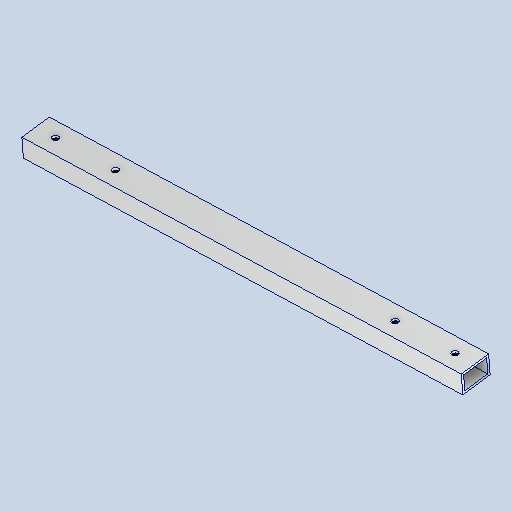
# Autodesk Inventor part: left_ASP
Saved by Autodesk Inventor 2024 (Build 280153000, 153)
## iProperties
Created: 2023-10-26
Part Number: left_ASP
Material: アルミニウム 6061
Document SubType Name: Modeling
Designer: jwith
Density: 2.7 g/cm^3
Appearance: アルミニウム - フラット
Mass: 32.0101 g
Surface Area: 199.643 cm^2
Volume: 11.8556 cm^3
Author: jwith
Autodesk Inventor part; units mm, degrees
ref_plane "YZ Plane" through (0, 0, 0) normal (1, 0, 0) x (0, 1, 0)
ref_plane "XZ Plane" through (0, 0, 0) normal (0, 1, 0) x (-1, 0, 0)
ref_plane "XY Plane" through (0, 0, 0) normal (0, 0, 1) x (1, 0, 0)
sketch "スケッチ1" plane through (0, 0, 0) normal (0, 1, 0) x (-1, 0, 0)
  line L0 (0, 0) -> (-15, 0)
  line L1 (-15, 0) -> (-15, -10)
  line L2 (-15, -10) -> (0, -10)
  line L3 (0, -10) -> (0, 0)
  dimension "d0" = 15
  dimension "d1" = 10
  constraints: 8 end point, 2 parallel, 1 horizontal, 1 perpendicular
  measures "d0" distance of L1.end L2.end
  measures "d1" distance of L2.end L0.start
extrude "押し出し1" add sketch "スケッチ1" against normal blind 220
shell "シェル1" thickness 1.2 removed faces 2 at (10, 0, -3.3333) at (10, -220, -3.3333)
sketch "スケッチ2" plane through (0, 0, 0) normal (0, 0, 1) x (1, 0, 0)
  line L0 (0, 0) -> (15, 0) projected
  line L1 (15, 0) -> (15, -220) projected
  line L2 (15, -220) -> (0, -220) projected
  point P0 (7.5, -10)
  point P1 (7.5, 0)
  point P2 (7.5, -40)
  point P3 (7.5, -210)
  point P4 (7.5, -210)
  point P5 (7.5, -180)
  dimension "d5" = 10
  dimension "d6" = 7.5
  dimension "d7" = 7.5
  dimension "d8" = 30
  dimension "d9" = 10
  dimension "d10" = 7.5
  dimension "d11" = 30
  dimension "d12" = 7.5
  constraints: 1 coincident, 1 midpoint
  measures "d5" distance of point (7.5, 0) point (7.5, -10)
  measures "d6" distance from line of L1 point (7.5, -10)
  measures "d7" distance from line of L1 point (7.5, -40)
  measures "d8" distance of point (7.5, -10) point (7.5, -40)
  measures "d9" distance from line of L2 point (7.5, -210)
  measures "d10" distance from line of L1 point (7.5, -210)
  measures "d11" distance of point (7.5, -210) point (7.5, -180)
  measures "d12" distance from line of L1 point (7.5, -180)
hole "穴1" at (7.5, -10, 0) at (7.5, -40, 0) at (7.5, -210, 0) at (7.5, -180, 0) direction (0, 0, -1) diameter 3.2 end through all
